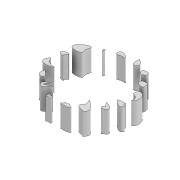
# Autodesk Inventor part: simple_ring4
Saved by Autodesk Inventor 2021 (Build 250183000, 183)
## iProperties
Created: 2022-04-12
Part Number: simple_ring4
Material: Generic
Document SubType Name: Modeling
Designer: Derm
Density: 1 g/cm^3
Appearance: Default
Author: Derm
Autodesk Inventor part; units mm, degrees
ref_plane "YZ Plane" through (0, 0, 0) normal (1, 0, 0) x (0, 1, 0)
ref_plane "XZ Plane" through (0, 0, 0) normal (0, 1, 0) x (-1, 0, 0)
ref_plane "XY Plane" through (0, 0, 0) normal (0, 0, 1) x (1, 0, 0)
sketch "Sketch1" plane through (0, 0, 0) normal (0, 1, 0) x (-1, 0, 0)
  line L0 (0, 0) -> (10000, 0)
  line L1 (0, 0) -> (9807.8528, -1950.9032) construction
  line L2 (-4839.2703, 7607.7402) -> (-3686.1301, 8453.7599) construction
  line L3 (-3686.1301, 8453.7599) -> (-5367.6765, 9477.4851) construction
  line L4 (-5367.6765, 9477.4851) -> (-6194.1579, 8840.6879) construction
  line L5 (-6194.1579, 8840.6879) -> (-6194.1579, 9938.1469) construction
  line L6 (-6194.1579, 9938.1469) -> (-6979.9927, 8718.748) construction
  line L7 (-6979.9927, 8718.748) -> (-7074.8348, 7865.1688) construction
  line L8 (-7074.8348, 7865.1688) -> (-6248.3534, 7350.3115) construction
  line L9 (-6248.3534, 7350.3115) -> (-3518.8943, 4626.9875) construction
  line L10 (-3518.8943, 4626.9875) -> (-5282.6353, 7062.3446) construction
  line L11 (-5282.6353, 7062.3446) -> (-4839.2703, 7607.7402) construction
  spline S0 degree 4 poles (-4839.2703, 7607.7402) (-3686.1301, 8453.7599) (-5367.6765, 9477.4851) (-6194.1579, 8840.6879) (-6194.1579, 9938.1469) (-6979.9927, 8718.748) (-7074.8348, 7865.1688) (-6248.3534, 7350.3115) (-3518.8943, 4626.9875) (-5282.6353, 7062.3446) (-4839.2703, 7607.7402) knots 1 1 1 1 1 2 3 4 5 6 7 8 8 8 8 8
  line L12 (-9368.0985, -3203.9118) -> (-8511.0158, -1632.5933) construction
  line L13 (-8511.0158, -1632.5933) -> (-10066.7098, -1632.5933) construction
  line L14 (-10066.7098, -1632.5933) -> (-10258.8207, -1293.8714) construction
  line L15 (-10258.8207, -1293.8714) -> (-10773.678, -386.0967) construction
  line L16 (-10773.678, -386.0967) -> (-10269.0249, 670.8774) construction
  line L17 (-10269.0249, 670.8774) -> (-11274.9864, -657.0742) construction
  line L18 (-11274.9864, -657.0742) -> (-11274.9864, -1402.2624) construction
  line L19 (-11274.9864, -1402.2624) -> (-10797.4408, -3203.9118) construction
  line L20 (-10797.4408, -3203.9118) -> (-9740.6089, -3203.9118) construction
  line L21 (-9740.6089, -3203.9118) -> (-9368.0985, -3203.9118) construction
  spline S1 degree 4 poles (-9368.0985, -3203.9118) (-8511.0158, -1632.5933) (-10066.7098, -1632.5933) (-10258.8207, -1293.8714) (-10773.678, -386.0967) (-10269.0249, 670.8774) (-11274.9864, -657.0742) (-11274.9864, -1402.2624) (-10797.4408, -3203.9118) (-9740.6089, -3203.9118) (-9368.0985, -3203.9118) knots 1 1 1 1 1 2 3 4 5 6 7 8 8 8 8 8
  line L22 (-4804.609, -8491.9009) -> (-4804.609, -7924.4901) construction
  line L23 (-4804.609, -7924.4901) -> (-5354.1276, -7924.4901) construction
  line L24 (-5354.1276, -7924.4901) -> (-5354.1276, -7119.8881) construction
  line L25 (-5354.1276, -7119.8881) -> (-6364.0042, -8076.8552) construction
  line L26 (-6364.0042, -8076.8552) -> (-6594.1987, -7924.4901) construction
  line L27 (-6594.1987, -7924.4901) -> (-6397.391, -8420.5803) construction
  line L28 (-6397.391, -8420.5803) -> (-6500.0442, -8936.6526) construction
  line L29 (-6500.0442, -8936.6526) -> (-5601.8884, -9094.8213) construction
  line L30 (-5601.8884, -9094.8213) -> (-4500.5485, -8799.9488) construction
  line L31 (-4500.5485, -8799.9488) -> (-4804.609, -8491.9009) construction
  spline S2 degree 4 poles (-4804.609, -8491.9009) (-4804.609, -7924.4901) (-5354.1276, -7924.4901) (-5354.1276, -7119.8881) (-6364.0042, -8076.8552) (-6594.1987, -7924.4901) (-6397.391, -8420.5803) (-6500.0442, -8936.6526) (-5601.8884, -9094.8213) (-4500.5485, -8799.9488) (-4804.609, -8491.9009) knots 1 1 1 1 1 2 3 4 5 6 7 8 8 8 8 8
  line L32 (8537.0831, 5074.1004) -> (8314.6961, 5236.4551) construction
  line L33 (8314.6961, 5236.4551) -> (8314.6961, 5249.669) construction
  line L34 (8314.6961, 5249.669) -> (7232.778, 6103.815) construction
  line L35 (7232.778, 6103.815) -> (7476.6578, 6605.1234) construction
  line L36 (7476.6578, 6605.1234) -> (8314.6961, 7025.1386) construction
  line L37 (8314.6961, 7025.1386) -> (9075.4251, 6225.7549) construction
  line L38 (9075.4251, 6225.7549) -> (9075.4251, 5656.7021) construction
  line L39 (9075.4251, 5656.7021) -> (9075.4251, 5074.1004) construction
  line L40 (9075.4251, 5074.1004) -> (8723.1543, 4626.9875) construction
  line L41 (8723.1543, 4626.9875) -> (8537.0831, 5074.1004) construction
  spline S3 degree 4 poles (8537.0831, 5074.1004) (8314.6961, 5236.4551) (8314.6961, 5249.669) (7232.778, 6103.815) (7476.6578, 6605.1234) (8314.6961, 7025.1386) (9075.4251, 6225.7549) (9075.4251, 5656.7021) (9075.4251, 5074.1004) (8723.1543, 4626.9875) (8537.0831, 5074.1004) knots 1 1 1 1 1 2 3 4 5 6 7 8 8 8 8 8
  line L42 (2531.318, 10954.3126) -> (2531.318, 10073.6357) construction
  line L43 (2531.318, 10073.6357) -> (2436.4759, 8786.4924) construction
  line L44 (2436.4759, 8786.4924) -> (1886.0734, 11555.3633) construction
  line L45 (1886.0734, 11555.3633) -> (1886.0734, 9322.6266) construction
  line L46 (1886.0734, 9322.6266) -> (878.3552, 10845.9216) construction
  line L47 (878.3552, 10845.9216) -> (1474.5057, 10954.3126) construction
  line L48 (1474.5057, 10954.3126) -> (1826.7765, 10629.1396) construction
  line L49 (1826.7765, 10629.1396) -> (2531.318, 10954.3126) construction
  spline S4 degree 4 poles (2531.318, 10954.3126) (2531.318, 10073.6357) (2436.4759, 8786.4924) (1886.0734, 11555.3633) (1886.0734, 9322.6266) (878.3552, 10845.9216) (1474.5057, 10954.3126) (1826.7765, 10629.1396) (2531.318, 10954.3126) knots 1 1 1 1 1 2 3 4 5 6 6 6 6 6
  line L50 (-1631.0559, -10907.6284) -> (-1631.0559, -9138.1703) construction
  line L51 (-1631.0559, -9138.1703) -> (-1777.6107, -8936.6526) construction
  line L52 (-1777.6107, -8936.6526) -> (-2732.1854, -7924.4901) construction
  line L53 (-2732.1854, -7924.4901) -> (-3568.9955, -10022.8993) construction
  line L54 (-3568.9955, -10022.8993) -> (-1631.0559, -10907.6284) construction
  spline S5 degree 4 poles (-1631.0559, -10907.6284) (-1631.0559, -9138.1703) (-1777.6107, -8936.6526) (-2732.1854, -7924.4901) (-3568.9955, -10022.8993) (-1631.0559, -10907.6284) knots 1 1 1 1 1 2 3 3 3 3 3
  line L55 (6238.4805, 8506.3447) -> (6238.4805, 9153.4105) construction
  line L56 (6238.4805, 9153.4105) -> (5103.2076, 9260.7031) construction
  line L57 (5103.2076, 9260.7031) -> (4785.0565, 8291.9584) construction
  line L58 (4785.0565, 8291.9584) -> (4021.3423, 8113.562) construction
  line L59 (4021.3423, 8113.562) -> (3760.7322, 7762.228) construction
  line L60 (3760.7322, 7762.228) -> (3686.2076, 7215.1404) construction
  line L61 (3686.2076, 7215.1404) -> (6973.7122, 9430.064) construction
  line L62 (6973.7122, 9430.064) -> (4389.4164, 6591.3632) construction
  line L63 (4389.4164, 6591.3632) -> (5484.1105, 7264.4944) construction
  line L64 (5484.1105, 7264.4944) -> (6565.6616, 7865.1688) construction
  line L65 (6565.6616, 7865.1688) -> (6486.4621, 8580.8185) construction
  line L66 (6486.4621, 8580.8185) -> (6238.4805, 8506.3447) construction
  spline S6 degree 4 poles (6238.4805, 8506.3447) (6238.4805, 9153.4105) (5103.2076, 9260.7031) (4785.0565, 8291.9584) (4021.3423, 8113.562) (3760.7322, 7762.228) (3686.2076, 7215.1404) (6973.7122, 9430.064) (4389.4164, 6591.3632) (5484.1105, 7264.4944) (6565.6616, 7865.1688) (6486.4621, 8580.8185) (6238.4805, 8506.3447) knots 1 1 1 1 1 2 3 4 5 6 7 8 9 10 10 10 10 10
  line L67 (-10258.8207, 1567.5332) -> (-7472.4395, 1567.5332) construction
  line L68 (-7472.4395, 1567.5332) -> (-9243.9564, 2541.5805) construction
  line L69 (-9243.9564, 2541.5805) -> (-9927.0456, 3577.9918) construction
  line L70 (-9927.0456, 3577.9918) -> (-11274.9864, 2806.0191) construction
  line L71 (-11274.9864, 2806.0191) -> (-10773.678, 2051.934) construction
  line L72 (-10773.678, 2051.934) -> (-10377.654, 2428.9766) construction
  line L73 (-10377.654, 2428.9766) -> (-10258.8207, 1567.5332) construction
  spline S7 degree 4 poles (-10258.8207, 1567.5332) (-7472.4395, 1567.5332) (-9243.9564, 2541.5805) (-9927.0456, 3577.9918) (-11274.9864, 2806.0191) (-10773.678, 2051.934) (-10377.654, 2428.9766) (-10258.8207, 1567.5332) knots 1 1 1 1 1 2 3 4 5 5 5 5 5
  spline S8 degree 5 poles (10355.9276, -5999.0073) (10836.7851, -5482.7997) (11276.6045, -4594.4755) (10342.4565, -3673.6348) (6110.1, -4678.2889) (9600.7935, -4903.2902) (6658.1105, -7937.3204) (8600.5149, -7408.6301) (9842.4202, -6550.265) (10355.9276, -5999.0073) knots 0 0 0 0 0 0 0.235647 0.386768 0.586768 0.748353 1 1 1 1 1 1
  spline S9 degree 5 poles (-8613.7447, -6122.8909) (-8367.8355, -6280.3663) (-7719.9799, -6374.981) (-6220.6993, -5975.5134) (-7267.3901, -4525.2396) (-9436.3113, -4483.4586) (-8781.0926, -5074.5218) (-8961.3802, -5706.0626) (-8797.6161, -6005.1433) (-8613.7447, -6122.8909) knots 0 0 0 0 0 0 0.276615 0.441741 0.641741 0.793169 1 1 1 1 1 1
  spline S10 degree 5 poles (5670.844, -8491.9009) (5742.2638, -8474.8774) (5806.4989, -8383.6279) (5683.4326, -8049.9151) (5430.923, -7278.7734) (5412.2868, -8156.0995) (5120.8, -8313.2914) (5433.0673, -8476.8737) (5602.6901, -8508.146) (5670.844, -8491.9009) knots 0 0 0 0 0 0 0.241164 0.402116 0.602116 0.769864 1 1 1 1 1 1
  spline S11 degree 4 poles (-1331.2246, 10276.4436) (-1844.122, 10901.3627) (-1177.8457, 8402.6007) (-2149.1474, 10889.2429) (-2679.562, 9128.661) (-3030.2367, 9999.2657) (-4156.4755, 10062.652) (-3479.9867, 10512.3604) (-2643.5785, 10663.2007) (-2011.1358, 10571.6481) (-891.5368, 10817.6263) (-1331.2246, 10276.4436) knots 0 0 0 0 0 0.203679 0.297412 0.393941 0.484079 0.575495 0.669142 0.766019 1 1 1 1 1
  spline S12 degree 5 poles (-8314.6961, 5198.8536) (-8302.6398, 5277.9236) (-8107.6964, 5310.843) (-7463.6703, 5225.9568) (-8300.4838, 6928.5402) (-8526.5466, 5667.0466) (-9541.5458, 5764.542) (-9303.8985, 4744.143) (-9164.9552, 4775.4566) (-6318.2906, 3170.4414) (-7981.9307, 4661.8848) (-8333.2809, 5076.9674) (-8314.6961, 5198.8536) knots 0 0 0 0 0 0 0.125579 0.214859 0.323214 0.437355 0.560081 0.6957 0.80642 1 1 1 1 1 1
  spline S13 degree 5 poles (9351.7652, -2315.8498) (9403.1239, -2142.7159) (9741.8684, -1760.5436) (10601.7831, -1121.2238) (8364.835, -1115.1568) (12074.5906, -1219.5798) (11022.481, -2543.7829) (9517.1072, -2727.8104) (9291.8488, -2517.8327) (9351.7652, -2315.8498) knots 0 0 0 0 0 0 0.224717 0.382113 0.582113 0.737839 1 1 1 1 1 1
  spline S14 degree 5 poles (10997.4506, 1076.3286) (11214.011, 1137.8062) (11754.6631, 1956.3506) (12900.2513, 4750.8844) (4133.4009, 1630.5105) (10778.196, 3411.3438) (10646.204, 1477.6252) (10816.0472, 1024.8314) (10997.4506, 1076.3286) knots 0 0 0 0 0 0 0.326503 0.526503 0.726503 1 1 1 1 1 1
  spline S15 degree 5 poles (2490.9307, -10280.177) (2856.1487, -10187.448) (3252.5618, -9627.9303) (2912.8466, -8020.3522) (1904.0339, -10508.0144) (-444.5065, -8263.0337) (1097.9466, -10058.3735) (2070.1634, -10387.0099) (2490.9307, -10280.177) knots 0 0 0 0 0 0 0.278798 0.478798 0.678798 1 1 1 1 1 1
  point P0 (9807.8528, 1950.9032)
  point P1 (8314.6961, 5555.7023)
  point P2 (5555.7023, 8314.6961)
  point P3 (1950.9032, 9807.8528)
  point P4 (-1950.9032, 9807.8528)
  point P5 (-5555.7023, 8314.6961)
  point P6 (-8314.6961, 5555.7023)
  point P7 (-9807.8528, 1950.9032)
  point P8 (-9807.8528, -1950.9032)
  point P9 (-8314.6961, -5555.7023)
  point P10 (-5555.7023, -8314.6961)
  point P11 (-1950.9032, -9807.8528)
  point P12 (1950.9032, -9807.8528)
  point P13 (5555.7023, -8314.6961)
  point P14 (8314.6961, -5555.7023)
  point P15 (9154.6321, -1820.9695)
  point P16 (7876.3496, -4624.774)
  point P17 (8089.7225, -5378.2949)
  point P18 (7895.6769, -7119.8881)
  point P19 (-7760.744, -4786.6795)
  point P20 (-8914.4109, -4775.9345)
  point P21 (-8914.4109, -5378.2949)
  point P22 (5484.1105, -7684.7756)
  point P23 (5325.8324, -8076.8552)
  point P24 (5325.8324, -8376.6104)
  point P25 (-1582.2435, 10159.7078)
  point P26 (-1658.8525, 9612.9733)
  point P27 (-2193.0943, 9950.2632)
  point P28 (-2673.2449, 9572.4274)
  point P29 (-3191.3093, 9848.2369)
  point P30 (-3812.2129, 10165.6403)
  point P31 (-3568.9955, 10405.583)
  point P32 (-2916.4851, 10591.3455)
  point P33 (-2212.585, 10629.1396)
  point P34 (-1326.4343, 10629.1399)
  point P35 (-8123.5987, 6181.6268)
  point P36 (-8631.0724, 5989.99)
  point P37 (-9243.9564, 5519.5703)
  point P38 (-9328.7655, 5074.1004)
  point P39 (-8852.8938, 4579.5664)
  point P40 (-7472.4395, 4055.4596)
  point P41 (9706.617, -1171.9315)
  point P42 (10863.6676, -1484.1264)
  point P43 (10363.5607, -2458.2081)
  point P44 (8220.7484, 2806.0191)
  point P45 (10549.8145, 1779.1903)
  point P46 (1713.9766, -9248.6798)
  point P47 (581.9894, -9248.6798)
  dimension "d1" = 11.25
  dimension "d4" = 360
  constraints: 11 vertical, 4 end point, 4 horizontal, 2 coincident, 1 point on line, 83 other
  measures "d1" angle of L1 L0
extrude "Extrusion2" add sketch "Sketch1" along normal blind 3000
mirror "Mirror1" about plane through (-1404.0276, 0, -9264.1833) normal (0, -1, 0) of "Extrusion2"
body "Solid2"
